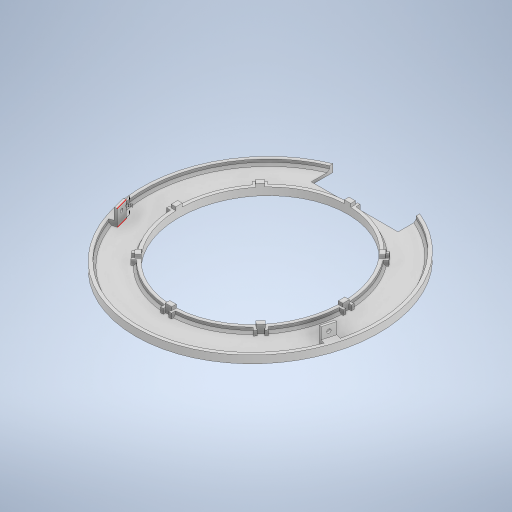
# Autodesk Inventor part: tampa_anel
Saved by Autodesk Inventor 2024.3 (Build 283343000, 343)
## iProperties
Created: 2024-12-01
Part Number: tampa_anel
Material: Genérico
Document SubType Name: Modeling
Designer: lostv
Density: 1 g/cm^3
Appearance: Padrão
Author: lostv
Autodesk Inventor part; units mm, degrees
ref_plane "YZ Plane" through (0, 0, 0) normal (1, 0, 0) x (0, 1, 0)
ref_plane "XZ Plane" through (0, 0, 0) normal (0, 1, 0) x (-1, 0, 0)
ref_plane "XY Plane" through (0, 0, 0) normal (0, 0, 1) x (1, 0, 0)
sketch "Esboço1" plane through (0, 0, 0) normal (0, 1, 0) x (-1, 0, 0)
  ellipse E0 centre (-0.1049, 6.8649) end of major axis (74.8951, 6.8649) minor radius 80.5 (74.8951, 6.8649) -> (-0.1049, 87.3649) ccw
  line L0 (-0.1049, 87.3649) -> (-0.1049, 6.8649)
  line L1 (-0.1049, 6.8649) -> (74.8951, 6.8649)
  line L2 (-0.1049, 6.8649) -> (54.7695, 61.7393)
  line L3 (-0.1049, 6.8649) -> (77.4993, 6.8649) construction
  line L4 (74.8951, 6.8649) -> (77.8951, 6.8649)
  ellipse E1 centre (-0.1049, 6.8649) end of major axis (-0.1049, 90.3649) minor radius 78 (53.6601, 67.3589) -> (4.8951, 90.1931) ccw
  ellipse E2 centre (-0.1049, 6.8649) end of major axis (-0.1049, 90.3649) minor radius 78 (77.7551, 11.8649) -> (60.2147, 59.8043) ccw
  ellipse E3 centre (-0.1049, 6.8649) end of major axis (-0.1049, 90.3649) minor radius 78 (-5.1049, 90.1931) -> (-53.87, 67.3589) ccw
  ellipse E4 centre (-0.1049, 6.8649) end of major axis (-75.1049, 6.8649) minor radius 80.5 (-0.1049, 87.3649) -> (-75.1049, 6.8649) ccw
  line L5 (-0.1049, 6.8649) -> (-54.9794, 61.7393)
  line L6 (-0.1049, 6.8649) -> (-75.1049, 6.8649) construction
  line L7 (-0.1049, 6.8649) -> (-75.1049, 6.8649)
  ellipse E5 centre (-0.1049, 6.8649) end of major axis (-0.1049, 90.3649) minor radius 78 (-60.4246, 59.8043) -> (-77.965, 11.8649) ccw
  line L8 (-79.3289, 9.8649) -> (-75.0528, 9.8649)
  line L9 (74.8951, 6.8649) -> (-75.1049, 6.8649)
  line L10 (-0.1049, 6.8649) -> (54.7695, -48.0096)
  ellipse E6 centre (-0.1049, 6.8649) end of major axis (74.8951, 6.8649) minor radius 80.5 (-0.1049, -73.6351) -> (74.8951, 6.8649) ccw
  line L11 (-0.1049, -73.6351) -> (-0.1049, 6.8649)
  line L12 (2.8951, -77.8529) -> (2.8951, -73.5707)
  line L13 (4.8951, -77.8529) -> (4.8951, -73.4561)
  line L14 (2.8951, -73.5707) -> (2.8951, -77.8529)
  ellipse E7 centre (-0.1049, 6.8649) end of major axis (-0.1049, -76.6351) minor radius 78 (4.8951, -76.4634) -> (53.6601, -53.6292) ccw
  ellipse E8 centre (-0.1049, 6.8649) end of major axis (-0.1049, -76.6351) minor radius 78 (60.2147, -46.0746) -> (77.7551, 1.8649) ccw
  line L15 (-53.0256, -50.1776) -> (-56.1839, -53.0214)
  line L16 (-56.9549, -45.6417) -> (-60.1987, -48.5625)
  line L17 (-56.9549, -45.6417) -> (-60.1987, -48.5625)
  line L18 (-53.0256, -50.1776) -> (-56.1839, -53.0214)
  line L19 (-3.1049, -77.8529) -> (-3.1049, -73.5707)
  line L20 (-3.1049, -73.5707) -> (-3.1049, -77.8529)
  line L21 (-5.1049, -77.8529) -> (-5.1049, -73.4561)
  ellipse E9 centre (-0.1049, 6.8649) end of major axis (-0.1049, -76.6351) minor radius 78 (-53.87, -53.6292) -> (-5.1049, -76.4634) ccw
  line L22 (-0.1049, 6.8649) -> (-54.9794, -48.0096)
  ellipse E10 centre (-0.1049, 6.8649) end of major axis (-75.1049, 6.8649) minor radius 80.5 (-75.1049, 6.8649) -> (-0.1049, -73.6351) ccw
  ellipse E11 centre (-0.1049, 6.8649) end of major axis (-0.1049, -76.6351) minor radius 78 (-77.965, 1.8649) -> (-60.4246, -46.0746) ccw
  line L23 (-79.3289, 3.8649) -> (-75.0818, 3.8649)
  line L24 (39.8951, -115.1529) -> (-40.1049, -115.1529)
  line L25 (-40.1049, -115.1529) -> (-40.1049, -115.1529)
  line L26 (-0.1049, -115.1529) -> (-0.1049, -121.655) construction
  line L27 (-79.3289, 1.8649) -> (-74.9601, 1.8649)
  line L28 (-79.3289, 11.8649) -> (-74.9601, 11.8649)
  line L29 (-79.3289, 1.8649) -> (-81.6289, 1.8649) construction
  line L30 (-81.6289, 1.8649) -> (-81.6289, 4.3649) construction
  line L31 (-81.6289, 4.3649) -> (-79.3289, 4.3649) construction
  line L32 (-79.3289, 1.8649) -> (-81.6289, 1.8649)
  line L33 (-81.6289, 4.3649) -> (-81.6289, 1.8649)
  line L34 (-81.6289, 4.3649) -> (-79.3289, 4.3649)
  line L35 (-79.3289, 4.3649) -> (-79.3289, 3.8649)
  line L36 (-79.3289, 9.8649) -> (-79.3289, 9.3649)
  line L37 (-81.6289, 9.3649) -> (-79.3289, 9.3649)
  line L38 (-81.6289, 9.3649) -> (-81.6289, 11.8649)
  line L39 (-81.6289, 11.8649) -> (-79.3289, 11.8649)
  line L40 (-79.3289, 3.8649) -> (-79.3289, 4.3649) construction
  line L41 (-79.3289, 9.3649) -> (-79.3289, 9.8649) construction
  line L42 (-79.3289, 4.3649) -> (-79.3289, 9.3649)
  line L43 (-56.1839, -53.0214) -> (-60.1987, -48.5625) construction
  line L44 (-61.537, -47.0762) -> (-58.1891, -44.0618)
  line L45 (-54.8457, -54.5077) -> (-51.6398, -51.6211)
  line L46 (-54.8457, -54.5077) -> (-56.5549, -56.0467)
  line L47 (-56.5549, -56.0467) -> (-58.2277, -54.1888)
  line L48 (-58.2277, -54.1888) -> (-56.5185, -52.6498)
  line L49 (-56.1839, -53.0214) -> (-56.5185, -52.6498)
  line L50 (-60.1987, -48.5625) -> (-56.5185, -52.6498)
  line L51 (-61.537, -47.0762) -> (-63.2462, -48.6152)
  line L52 (-63.2462, -48.6152) -> (-61.5734, -50.4731)
  line L53 (-61.5734, -50.4731) -> (-59.8642, -48.9341)
  line L54 (2.8951, -77.8529) -> (-3.1049, -77.8529) construction
  line L55 (-5.1049, -77.8529) -> (-5.1049, -80.1529)
  line L56 (-5.1049, -80.1529) -> (-2.6049, -80.1529)
  line L57 (-2.6049, -80.1529) -> (-2.6049, -77.8529)
  line L58 (-3.1049, -77.8529) -> (-2.6049, -77.8529)
  line L59 (4.8951, -77.8529) -> (4.8951, -80.1529)
  line L60 (4.8951, -80.1529) -> (2.3951, -80.1529)
  line L61 (2.3951, -80.1529) -> (2.3951, -77.8529)
  line L62 (2.8951, -77.8529) -> (2.3951, -77.8529)
  line L63 (-2.6049, -77.8529) -> (2.3951, -77.8529)
  line L64 (63.0363, -48.6152) -> (61.3635, -50.4731)
  line L65 (61.3271, -47.0762) -> (63.0363, -48.6152)
  line L66 (61.3635, -50.4731) -> (59.6543, -48.9341)
  line L67 (56.745, -45.6417) -> (59.9888, -48.5625)
  line L68 (61.3271, -47.0762) -> (57.9792, -44.0618)
  line L69 (59.9888, -48.5625) -> (56.3086, -52.6498)
  line L70 (55.9741, -53.0214) -> (59.9888, -48.5625) construction
  line L71 (52.8157, -50.1776) -> (55.9741, -53.0214)
  line L72 (55.9741, -53.0214) -> (56.3086, -52.6498)
  line L73 (58.0178, -54.1888) -> (56.3086, -52.6498)
  line L74 (56.345, -56.0467) -> (58.0178, -54.1888)
  line L75 (54.6358, -54.5077) -> (56.345, -56.0467)
  line L76 (54.6358, -54.5077) -> (51.4299, -51.6211)
  line L77 (79.119, 1.8649) -> (81.419, 1.8649)
  line L78 (81.419, 1.8649) -> (81.419, 4.3649)
  line L79 (81.419, 4.3649) -> (79.119, 4.3649)
  line L80 (79.119, 4.3649) -> (79.119, 3.8649)
  line L81 (79.119, 3.8649) -> (74.8719, 3.8649)
  line L82 (79.119, 1.8649) -> (74.7502, 1.8649)
  line L83 (79.119, 4.3649) -> (79.119, 9.3649)
  line L84 (81.419, 9.3649) -> (79.119, 9.3649)
  line L85 (79.119, 9.8649) -> (79.119, 9.3649)
  line L86 (81.419, 9.3649) -> (81.419, 11.8649)
  line L87 (81.419, 11.8649) -> (79.119, 11.8649)
  line L88 (79.119, 11.8649) -> (74.7502, 11.8649)
  line L89 (79.119, 9.8649) -> (74.843, 9.8649)
  line L90 (55.9741, 66.7511) -> (56.3086, 66.3796)
  line L91 (54.6358, 68.2374) -> (56.345, 69.7764)
  line L92 (56.345, 69.7764) -> (58.0178, 67.9186)
  line L93 (58.0178, 67.9186) -> (56.3086, 66.3796)
  line L94 (55.9741, 66.7511) -> (59.9888, 62.2923) construction
  line L95 (59.9888, 62.2923) -> (56.3086, 66.3796)
  line L96 (61.3635, 64.2028) -> (59.6543, 62.6638)
  line L97 (63.0363, 62.345) -> (61.3635, 64.2028)
  line L98 (61.3271, 60.806) -> (63.0363, 62.345)
  line L99 (61.3271, 60.806) -> (57.9792, 57.7915)
  line L100 (56.745, 59.3715) -> (59.9888, 62.2923)
  line L101 (52.8157, 63.9073) -> (55.9741, 66.7511)
  line L102 (54.6358, 68.2374) -> (51.4299, 65.3508)
  line L103 (-54.8457, 68.2374) -> (-51.6398, 65.3508)
  line L104 (-54.8457, 68.2374) -> (-56.5549, 69.7764)
  line L105 (-56.5549, 69.7764) -> (-58.2277, 67.9186)
  line L106 (-58.2277, 67.9186) -> (-56.5185, 66.3796)
  line L107 (-56.1839, 66.7511) -> (-56.5185, 66.3796)
  line L108 (-53.0256, 63.9073) -> (-56.1839, 66.7511)
  line L109 (-60.1987, 62.2923) -> (-56.5185, 66.3796)
  line L110 (-61.5734, 64.2028) -> (-59.8642, 62.6638)
  line L111 (-56.9549, 59.3715) -> (-60.1987, 62.2923)
  line L112 (-63.2462, 62.345) -> (-61.5734, 64.2028)
  line L113 (-61.537, 60.806) -> (-63.2462, 62.345)
  line L114 (-61.537, 60.806) -> (-58.1891, 57.7915)
  line L115 (-5.1049, 91.5826) -> (-5.1049, 93.8826)
  line L116 (-5.1049, 91.5826) -> (-5.1049, 87.1858)
  line L117 (-5.1049, 93.8826) -> (-2.6049, 93.8826)
  line L118 (-2.6049, 93.8826) -> (-2.6049, 91.5826)
  line L119 (-3.1049, 91.5826) -> (-2.6049, 91.5826)
  line L120 (-3.1049, 91.5826) -> (-3.1049, 87.3004)
  line L121 (-2.6049, 91.5826) -> (2.3951, 91.5826)
  line L122 (2.3951, 93.8826) -> (2.3951, 91.5826)
  line L123 (4.8951, 93.8826) -> (2.3951, 93.8826)
  line L124 (4.8951, 91.5826) -> (4.8951, 87.1858)
  line L125 (4.8951, 91.5826) -> (4.8951, 93.8826)
  line L126 (2.8951, 91.5826) -> (2.8951, 87.3004)
  line L127 (2.8951, 91.5826) -> (-3.1049, 91.5826) construction
  line L128 (2.8951, 91.5826) -> (2.3951, 91.5826)
  line L129 (74.8719, 3.8649) -> (74.843, 3.8649)
  line L130 (-75.0818, 3.8649) -> (-75.0528, 3.8649)
  line L131 (-40.1049, -115.1529) -> (39.8951, -115.1529)
  line L132 (39.8951, -115.1529) -> (39.8951, -80.1529)
  line L133 (-40.1049, -80.1529) -> (-40.1049, -115.1529)
  line L134 (-0.1049, 6.8649) -> (-0.1049, 118.8649) construction
  line L135 (-0.1049, 6.8649) -> (106.3951, 6.8649) construction
  line L136 (-0.1049, 6.8649) -> (-0.1049, -101.6351) construction
  line L137 (-0.1049, 6.8649) -> (-106.6049, 6.8649) construction
  line L138 (-0.1049, 6.8649) -> (109.3951, 6.8649) construction
  line L139 (-0.1049, 6.8649) -> (-109.6049, 6.8649) construction
  line L140 (-0.1049, 6.8649) -> (-0.1049, 121.8649) construction
  line L141 (-0.1049, 6.8649) -> (-0.1049, -104.6351) construction
  line L142 (2.3951, -80.1529) -> (2.3951, -77.8529)
  line L143 (-2.6049, -77.8529) -> (-2.6049, -80.1529)
  line L144 (-2.6049, -77.8529) -> (2.3951, -77.8529)
  line L145 (39.8951, -80.1529) -> (2.3951, -80.1529)
  line L146 (-2.6049, -80.1529) -> (-40.1049, -80.1529)
  ellipse E12 centre (-0.1049, 6.8649) end of major axis (109.3951, 6.8649) minor radius 115 (39.8951, -100.1876) -> (-40.1049, -100.1876) ccw
  line L147 (98.2829, 34.7328) -> (95.1718, 46.1212)
  line L148 (95.1718, 46.1212) -> (99.2372, 47.2318)
  line L149 (98.2829, 34.7328) -> (102.7411, 35.9507)
  line L150 (-98.4928, 34.7328) -> (-102.951, 35.9507)
  line L151 (-98.4928, 34.7328) -> (-95.3817, 46.1212)
  line L152 (-95.3817, 46.1212) -> (-99.4471, 47.2318)
  ellipse E13 centre (-0.1049, 6.8649) end of major axis (106.3951, 6.8649) minor radius 112 (39.8951, -96.9353) -> (102.7411, 35.9507) ccw
  ellipse E14 centre (-0.1049, 6.8649) end of major axis (106.3951, 6.8649) minor radius 112 (99.2372, 47.2318) -> (-99.4471, 47.2318) ccw
  ellipse E15 centre (-0.1049, 6.8649) end of major axis (106.3951, 6.8649) minor radius 112 (-102.951, 35.9507) -> (-40.1049, -96.9353) ccw
  circle A0 centre (32.8951, -87.1529) radius 1.75
  circle A1 centre (-33.1049, -87.1529) radius 1.75
  point P0 (0, 0)
  point P1 (94.8951, 6.8649)
  point P2 (97.8951, 6.8649)
  point P3 (-84.0674, 6.8649)
  point P4 (-55.6386, -52.5304)
  point P5 (-80.4789, 4.3649)
  point P6 (-80.4789, 1.8649)
  point P7 (-79.3289, 4.1149)
  point P8 (-79.3289, 9.6149)
  point P9 (-80.4789, 11.8649)
  point P10 (-77.1445, 11.8649)
  point P11 (-55.7003, -55.2772)
  point P12 (-60.7188, -49.7036)
  point P13 (-62.4098, -49.5442)
  point P14 (2.3951, -79.0029)
  point P15 (-2.8549, -77.8529)
  point P16 (2.8951, -75.7118)
  point P17 (79.119, 4.1149)
  point P18 (-79.3289, 6.8649)
  point P19 (-41.5382, -96.5651)
  point P20 (41.3283, -96.5651)
  point P21 (39.8951, -94.138)
  point P22 (3.6451, 93.8826)
  point P23 (81.419, 3.1149)
  point P24 (-5.1049, 90.1931)
  point P25 (77.7551, 1.8649)
  dimension "d3" = 83.5
  dimension "d4" = 78
  dimension "d0" = 75
  dimension "d1" = 80.5
  dimension "d2" = 45
  dimension "d5" = 2.5
  dimension "d6" = 2
  dimension "d7" = 2.3
  dimension "d8" = 2.3
  dimension "d9" = 2
  dimension "d10" = 2.5
  dimension "d11" = 6.6688
  dimension "d12" = 2.5
  dimension "d13" = 2.5
  dimension "d14" = 2.3
  dimension "d15" = 2.5
  dimension "d16" = 2.5
  dimension "d17" = 2.3
  dimension "d18" = 4.2822
  dimension "d19" = 6
  dimension "d20" = 112
  dimension "d21" = 106.5
  dimension "d22" = 106.5
  dimension "d23" = 109.5
  dimension "d24" = 109.5
  dimension "d25" = 115
  dimension "d26" = 24.9822
  dimension "d27" = 24.9761
  dimension "d28" = 80
  dimension "d29" = 40
  dimension "d30" = 35
  dimension "d31" = 3.5
  dimension "d32" = 7
  dimension "d33" = 7
  constraints: 306 end point, 100 symmetric about line, 47 point on line, 21 perpendicular, 17 horizontal, 16 midpoint, 15 coincident, 12 collinear, 12 vertical, 4 parallel, 2 centre point, 1 equal length, 105 other
  measures "d0" distance of L11.end L9.start
  measures "d1" distance of L0.start L11.end
  measures "d2" angle of L3 L2
  measures "d5" distance of point (-80.479, 4.365) point (-80.479, 1.865)
  measures "d6" distance between parallel lines of L27 L23
  measures "d7" distance from line of point (-79.329, 4.115) L33
  measures "d8" distance from line of point (-79.329, 9.615) L38
  measures "d9" distance from line of L8 point (-77.145, 11.865)
  measures "d10" distance from line of point (-80.479, 11.865) L37
  measures "d11" distance of L27.end L29.end
  measures "d12" distance from line of point (-55.7, -55.277) L48
  measures "d13" distance from line of point (-60.719, -49.704) L51
  measures "d14" distance between parallel lines of L43 L52
  measures "d15" distance between parallel lines of L57 L55
  measures "d16" distance from line of L59 point (2.395, -79.003)
  measures "d17" distance from line of point (-2.855, -77.853) L56
  measures "d18" distance of L19.start L19.end
  measures "d19" distance from line of point (2.895, -75.712) L19
  measures "d20" distance of L136.start L134.end
  measures "d21" distance of L136.start L135.end
  measures "d22" distance of L136.start L137.end
  measures "d23" distance of L141.start L138.end
  measures "d24" distance of L141.start L139.end
  measures "d25" distance of L141.start L140.end
  measures "d26" vertical distance of point (3.645, 93.883) L134.end
  measures "d27" horizontal distance of point (81.419, 3.115) L135.end
  measures "d28" distance between parallel lines of L132 L133
  measures "d29" distance between parallel lines of L136 L132
  measures "d30" distance of L133.start L25.end
  measures "d31" diameter of A0
  measures "d32" distance from line of L132 A0.centre
  measures "d33" distance from line of L145 A0.centre
extrude "Extrusão1" add sketch "Esboço1" along normal blind 2.5 contours E2 L99 L98 L97 L96 L95 L93 L92 L91 L102 E1 L124 L125 L123 L122 L121 L118 L117 L115 L116 E3 L103 L104 L105 L106 L109 L110 L112 L113 L114 E5 L28 L39 L38 L37 L42 L34 L33 L32 L27 E11 L44 L51 L52 L53 L50 L48 L47 L46 L45 E9 L21 L55 L146 L133 E15 L150 L151 L152 E14 L148 L147 L149 E13 L132 L145 L59 L13 E7 L76 L75 L74 L73 L69 L66 L64 L65 L68 E8 L82 L77 L78 L79 L83 L84 L86 L87 L88
extrude "Extrusão2" add sketch "Esboço1" along normal blind 7 contours E0 L88 L87 L86 L84 L85 L89 | L129 L81 L80 L79 L78 L77 L82 E6 | E0 L99 E2 L88 | L82 E8 L68 E6 | E0 L100 L95 L96 L97 L98 L99 | L126 L128 L122 L123 L125 L124 E0 | E4 L116 L115 L117 L118 L119 L120 | E0 L102 L91 L92 L93 L90 L101 | L108 L107 L106 L105 L104 L103 E4 | E4 L114 L113 L112 L110 L109 L111 | L8 L36 L37 L38 L39 L28 E4 | E10 L27 L32 L33 L34 L35 L23 L130 | L71 L72 L73 L74 L75 L76 E6 | E6 L68 L65 L64 L66 L69 L67 | E6 L13 L59 L60 L61 L62 L12 | L19 L58 L57 L56 L55 L21 E10 | L16 L50 L53 L52 L51 L44 E10 | E10 L45 L46 L47 L48 L49 L15 | L124 E1 L102 E0 | E4 L103 E3 L116 | E4 L28 E5 L114 | E10 L44 E11 L27 | L76 E7 L13 E6 | L21 E9 L45 E10 | E13 L149 L147 L148 E14 L152 L151 L150 E15 L133 E12 L132
extrude "Extrusão3" add sketch "Esboço1" along normal blind 10 contours E0 L89 L85 L83 L80 L81 L129 E6 | E4 L120 L119 L121 L128 L126 E0 | E0 L101 L90 L95 L100 | E4 L111 L109 L107 L108 | E10 L130 L23 L35 L42 L36 L8 E4 | E6 L67 L69 L72 L71 | E6 L12 L62 L63 L58 L19 E10 | E10 L15 L49 L50 L16
sketch "Esboço2" plane through (0, 2.5, 0) normal (0, 1, 0) x (1, 0, 0)
  line L0 (95.3817, -46.1212) -> (98.4928, -34.7328) projected
  line L1 (98.4928, -34.7328) -> (95.3817, -46.1212)
  line L2 (95.3817, -46.1212) -> (93.4524, -45.5941)
  line L3 (93.4524, -45.5941) -> (96.5635, -34.2058)
  line L4 (96.5635, -34.2058) -> (98.4928, -34.7328)
  line L5 (102.951, -35.9507) -> (98.4928, -34.7328) projected
  line L6 (95.3817, -46.1212) -> (99.4471, -47.2318) projected
  line L7 (-95.3671, -46.1745) -> (-98.4928, -34.7328)
  line L8 (-95.3671, -46.1745) -> (-93.2425, -45.5941)
  line L9 (-93.2425, -45.5941) -> (-96.3536, -34.2058)
  line L10 (-96.3536, -34.2058) -> (-98.4782, -34.7862)
  line L11 (-98.2829, -34.7328) -> (-102.7411, -35.9507) projected
  line L12 (-99.2372, -47.2318) -> (-95.1718, -46.1212) projected
  line L13 (-95.1718, -46.1212) -> (-98.2829, -34.7328) projected
  point P0 (0, 0)
  dimension "d40" = 2
  dimension "d43" = 2
  constraints: 16 end point, 5 collinear, 3 perpendicular, 2 point on line
  measures "d40" distance between parallel lines of L3 L0
  measures "d43" distance between parallel lines of L9 L13
extrude "Extrusão4" add sketch "Esboço2" along normal blind 15
sketch "Esboço3" plane through (-95.3671, 7, 46.1745) normal (-0.9647, 0, 0.2635) x (0.2635, 0, 0.9647)
  circle A0 centre (-5.9, 5) radius 1.75
  line L0 (0, 0) -> (0, 10.5) projected
  line L1 (101.866, 0) -> (-126.5701, 0) projected
  point P0 (-19.4105, -7)
  point P1 (-105.4879, 0)
  dimension "d44" = 3.5
  dimension "d45" = 5.9
  dimension "d46" = 5
  constraints: 1 centre point
  measures "d44" diameter of A0
  measures "d45" distance from line of L0 A0.centre
  measures "d46" distance from line of L1 A0.centre
extrude "Extrusão5" cut sketch "Esboço3" against normal blind 15
sketch "Esboço4" plane through (98.4928, 7, 34.7328) normal (0.9647, 0, 0.2635) x (0.2635, 0, -0.9647)
  circle A0 centre (-5.9, 5) radius 1.75
  line L0 (0, 0) -> (0, 10.5) projected
  line L1 (114.7644, 0) -> (-113.6716, 0) projected
  point P0 (7.5495, -7)
  point P1 (0, 5.25)
  point P2 (93.6822, 0)
  dimension "d49" = 3.5
  dimension "d50" = 5.9
  dimension "d51" = 5
  constraints: 1 centre point, 1 midpoint
  measures "d49" diameter of A0
  measures "d50" horizontal distance of point (0, 5.25) A0.centre
  measures "d51" distance from line of L1 A0.centre
extrude "Extrusão6" cut sketch "Esboço4" against normal blind 15
chamfer "Chanfro1" distance 2 angle 45 11 edges at (95.4621, 2.5, -43.0108) (0.1049, 2.5, 118.8649) (-72.5226, 2.5, 37.318) (-72.5226, 2.5, -23.5883) (-31.1533, 2.5, -69.6369) (31.3632, 2.5, -69.6369) (-31.1533, 2.5, 83.3666) (31.3632, 2.5, 83.3666) (72.7325, 2.5, 37.318) (-95.2522, 2.5, -43.0108) (72.7325, 2.5, -23.5883)
sketch "Esboço5" plane through (-96.3536, 2.5, 34.2058) normal (0.9647, 0, -0.2635) x (-0.2635, 0, -0.9647)
  line L0 (0, 0) -> (-11.8057, 0) projected
  line L1 (-11.8057, 15) -> (0, 15) projected
  point P0 (7.6048, -2.5)
  dimension "d57" = 15
  measures "d57" distance between parallel lines of L0 L1
